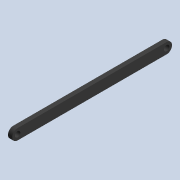
# Autodesk Inventor part: base3
Saved by Autodesk Inventor 2021 (Build 250183000, 183)
## iProperties
Part Number: base3
Material: Generic
Document SubType Name: Modeling
Designer: Dell
Appearance: Default
Author: Dell
Autodesk Inventor part; units mm, degrees
ref_plane "YZ Plane" through (0, 0, 0) normal (1, 0, 0) x (0, 1, 0)
ref_plane "XZ Plane" through (0, 0, 0) normal (0, 1, 0) x (-1, 0, 0)
ref_plane "XY Plane" through (0, 0, 0) normal (0, 0, 1) x (1, 0, 0)
sketch "Sketch1" plane through (0, 0, 0) normal (1, 0, 0) x (0, 1, 0)
  line L0 (0, 0) -> (0, -70)
  arc A0 (2.5, 0) -> (-2.5, 0) centre (0, 0) ccw
  arc A1 (-2.5, -70) -> (2.5, -70) centre (0, -70) ccw
  line L1 (2.5, 0) -> (2.5, -70)
  line L2 (-2.5, 0) -> (-2.5, -70)
  circle A2 centre (0, 0) radius 1.25
  circle A3 centre (0, -70) radius 1.25
  dimension "d0" = 70
  dimension "d1" = 5
  dimension "d2" = 5
  dimension "d3" = 2.5
  dimension "d4" = 2.5
  constraints: 6 end point, 4 centre point, 4 coincident, 4 point on circle, 2 tangent, 1 vertical
  measures "d0" distance of L0.start L0.end
  measures "d1" diameter of A0
  measures "d2" diameter of A1
  measures "d3" diameter of A2
  measures "d4" diameter of A3
extrude "Extrusion1" add sketch "Sketch1" along normal blind 2
body "Solid1"
